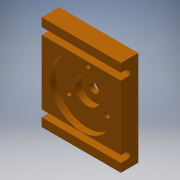
# Autodesk Inventor part: Fixation_moteur
Saved by Autodesk Inventor 2016 SP1 (Build 200210100, 210)
## iProperties
Created: 2016-01-21
Part Number: Fixation_moteur
Material: Plastique ABS
Document SubType Name: Modeling
Designer: sd
Density: 1.06 g/cm^3
Appearance: Orange
Mass: 25.9376 g
Surface Area: 102.342 cm^2
Volume: 24.4694 cm^3
Author: sd
Autodesk Inventor part; units mm, degrees
ref_plane "YZ Plane" through (0, 0, 0) normal (1, 0, 0) x (0, 1, 0)
ref_plane "XZ Plane" through (0, 0, 0) normal (0, 1, 0) x (-1, 0, 0)
ref_plane "XY Plane" through (0, 0, 0) normal (0, 0, 1) x (1, 0, 0)
sketch "Esquisse2" plane through (0, 0, 0) normal (0, 1, 0) x (-1, 0, 0)
  line L0 (25, -30) -> (-25, -30)
  line L1 (-25, -30) -> (-25, 30)
  line L2 (-25, 30) -> (25, 30)
  line L3 (25, 30) -> (25, -30)
  point P0 (0, 0)
  dimension "d0" = 50
  dimension "d1" = 60
  dimension "d2" = 25
  dimension "d3" = 30
  constraints: 8 end point, 2 parallel, 1 horizontal, 1 perpendicular
  measures "d0" distance of L0.start L0.end
  measures "d1" distance of L2.end L0.start
  measures "d2" horizontal distance of point (0, 0) L0.start
  measures "d3" vertical distance of L0.start point (0, 0)
extrude "Extrusion1" add sketch "Esquisse2" along normal blind 11
sketch "Esquisse3" plane through (25, 0, 30) normal (1, 0, 0) x (0, 0, -1)
  line L0 (60, 0) -> (0, 0) projected
  line L1 (60, 0) -> (60, 11) projected
  line L2 (0, 0) -> (0, 11) projected
  circle A0 centre (7.5, 4) radius 2.15
  circle A1 centre (52.5, 4) radius 2.15
  line L3 (5.35, 4) -> (5.35, 0)
  line L4 (9.65, 4) -> (9.65, 0)
  line L5 (9.65, 0) -> (5.35, 0)
  line L6 (50.35, 4) -> (50.35, 0)
  line L7 (54.65, 4) -> (54.65, 0)
  line L8 (54.65, 0) -> (50.35, 0)
  point P0 (30, 0)
  dimension "d6" = 4.3
  dimension "d7" = 4.3
  dimension "d8" = 45
  dimension "d9" = 7.5
  dimension "d10" = 7.5
  dimension "d11" = 60
  dimension "d12" = 4
  constraints: 12 end point, 4 perpendicular, 4 point on circle, 4 point on line, 4 tangent, 2 centre point, 2 collinear
  measures "d6" diameter of A0
  measures "d7" diameter of A1
  measures "d8" distance of A1.centre A0.centre
  measures "d9" distance from line of L2 A0.centre
  measures "d10" distance from line of L1 A1.centre
  measures "d11" distance of L2.end L1.end
  measures "d12" distance from line of L0 A0.centre
extrude "Extrusion2" cut sketch "Esquisse3" against normal through all
sketch "Esquisse4" plane through (0, 0, 0) normal (0, -1, 0) x (1, 0, 0)
  circle A0 centre (0, 0) radius 20
  dimension "d15" = 40
  constraints: 1 centre point, 1 coincident
  measures "d15" diameter of A0
extrude "Extrusion3" cut sketch "Esquisse4" against normal blind 4
sketch "Esquisse5" plane through (0, 4, 0) normal (0, -1, 0) x (1, 0, 0)
  circle A0 centre (0, 0) radius 20 projected
  circle A1 centre (0, 0) radius 8
  point P0 (8.7559, 17.9815)
  point P1 (8.7559, -17.9815)
  dimension "d18" = 16
  constraints: 1 centre point, 1 coincident
  measures "d18" diameter of A1
extrude "Extrusion4" cut sketch "Esquisse5" against normal blind 4 contours A1
sketch "Esquisse7" plane through (0, 8, 0) normal (0, -1, 0) x (1, 0, 0)
  circle A0 centre (0, 0) radius 8 projected
  circle A1 centre (0, 0) radius 3
  dimension "d24" = 6
  constraints: 1 centre point, 1 coincident
  measures "d24" diameter of A1
extrude "Extrusion6" cut sketch "Esquisse7" against normal through all contours A1
sketch "Esquisse8" plane through (0, 4, 0) normal (0, -1, 0) x (1, 0, 0)
  circle A0 centre (0, 0) radius 8 projected
  circle A1 centre (0, 14) radius 1.6
  dimension "d27" = 3.2
  dimension "d28" = 14
  constraints: 1 centre point
  measures "d27" diameter of A1
  measures "d28" distance of A1.centre A0.centre
extrude "Extrusion7" cut sketch "Esquisse8" against normal through all contours A1
pattern_circular "Réseau circulaire1" count 3 over 360 about axis through (0, 4, 0) along (0, 1, 0) of "Extrusion7"
equation "\"d2\" = 0.5 * d0"
equation "\"d3\" = 0.5 * d1"
equation "\"d9\" = d10"
equation "\"d10\" = -0.5 * d8 + 0.5 * d11"
